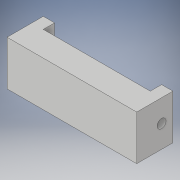
# Autodesk Inventor part: cap
Saved by Autodesk Inventor 2019 (Build 230136000, 136)
## iProperties
Created: 2019-05-07
Part Number: cap
Material: Generic
Document SubType Name: Modeling
Designer: Alex Jones
Density: 1 g/cm^3
Appearance: Default
Author: Alex Jones
Autodesk Inventor part; units mm, degrees
ref_plane "YZ Plane" through (0, 0, 0) normal (1, 0, 0) x (0, 1, 0)
ref_plane "XZ Plane" through (0, 0, 0) normal (0, 1, 0) x (-1, 0, 0)
ref_plane "XY Plane" through (0, 0, 0) normal (0, 0, 1) x (1, 0, 0)
sketch "Sketch1" plane through (0, 0, 0) normal (0, 0, 1) x (1, 0, 0)
  circle A0 centre (-40, 0) radius 2.5 projected
  arc A1 (-31.25, -10) -> (-30, -8.75) centre (-31.25, -8.75) ccw projected
  line L0 (-30, -3.6) -> (-30, -8.75) projected
  line L1 (-30.5, -3.1) -> (-30, -3.6) projected
  line L2 (-31.6, -3.1) -> (-30.5, -3.1) projected
  line L3 (-31.6, -5.5) -> (-31.6, -3.1) projected
  line L4 (-33.534, -5.5) -> (-31.6, -5.5) projected
  line L5 (-35.9, -3.134) -> (-33.534, -5.5) projected
  line L6 (-35.9, 3.134) -> (-35.9, -3.134) projected
  line L7 (-33.534, 5.5) -> (-35.9, 3.134) projected
  line L8 (-31.6, 5.5) -> (-33.534, 5.5) projected
  line L9 (-31.6, 3.1) -> (-31.6, 5.5) projected
  line L10 (-30.5, 3.1) -> (-31.6, 3.1) projected
  line L11 (-30, 3.6) -> (-30.5, 3.1) projected
  line L12 (-30, 8.75) -> (-30, 3.6) projected
  arc A2 (-30, 8.75) -> (-31.25, 10) centre (-31.25, 8.75) ccw projected
  line L13 (-36.4, 10) -> (-31.25, 10) projected
  line L14 (-36.9, 9.5) -> (-36.4, 10) projected
  line L15 (-36.9, 8.4) -> (-36.9, 9.5) projected
  line L16 (-34.5, 8.4) -> (-36.9, 8.4) projected
  line L17 (-34.5, 6.466) -> (-34.5, 8.4) projected
  line L18 (-36.866, 4.1) -> (-34.5, 6.466) projected
  line L19 (-43.134, 4.1) -> (-36.866, 4.1) projected
  line L20 (-45.5, 6.466) -> (-43.134, 4.1) projected
  line L21 (-45.5, 8.4) -> (-45.5, 6.466) projected
  line L22 (-43.1, 8.4) -> (-45.5, 8.4) projected
  line L23 (-43.1, 9.5) -> (-43.1, 8.4) projected
  line L24 (-43.6, 10) -> (-43.1, 9.5) projected
  line L25 (-48.75, 10) -> (-43.6, 10) projected
  arc A3 (-48.75, 10) -> (-50, 8.75) centre (-48.75, 8.75) ccw projected
  line L26 (-50, 3.6) -> (-50, 8.75) projected
  line L27 (-49.5, 3.1) -> (-50, 3.6) projected
  line L28 (-48.4, 3.1) -> (-49.5, 3.1) projected
  line L29 (-48.4, 5.5) -> (-48.4, 3.1) projected
  line L30 (-46.466, 5.5) -> (-48.4, 5.5) projected
  line L31 (-44.1, 3.134) -> (-46.466, 5.5) projected
  line L32 (-44.1, -3.134) -> (-44.1, 3.134) projected
  line L33 (-46.466, -5.5) -> (-44.1, -3.134) projected
  line L34 (-48.4, -5.5) -> (-46.466, -5.5) projected
  line L35 (-48.4, -3.1) -> (-48.4, -5.5) projected
  line L36 (-49.5, -3.1) -> (-48.4, -3.1) projected
  line L37 (-50, -3.6) -> (-49.5, -3.1) projected
  line L38 (-50, -8.75) -> (-50, -3.6) projected
  arc A4 (-50, -8.75) -> (-48.75, -10) centre (-48.75, -8.75) ccw projected
  line L39 (-43.6, -10) -> (-48.75, -10) projected
  line L40 (-43.1, -9.5) -> (-43.6, -10) projected
  line L41 (-43.1, -8.4) -> (-43.1, -9.5) projected
  line L42 (-45.5, -8.4) -> (-43.1, -8.4) projected
  line L43 (-45.5, -6.466) -> (-45.5, -8.4) projected
  line L44 (-43.134, -4.1) -> (-45.5, -6.466) projected
  line L45 (-36.866, -4.1) -> (-43.134, -4.1) projected
  line L46 (-34.5, -6.466) -> (-36.866, -4.1) projected
  line L47 (-34.5, -8.4) -> (-34.5, -6.466) projected
  line L48 (-36.9, -8.4) -> (-34.5, -8.4) projected
  line L49 (-36.9, -9.5) -> (-36.9, -8.4) projected
  line L50 (-36.4, -10) -> (-36.9, -9.5) projected
  line L51 (-31.25, -10) -> (-36.4, -10) projected
  circle A5 centre (0, 0) radius 2.5 projected
  arc A6 (8.75, -10) -> (10, -8.75) centre (8.75, -8.75) ccw projected
  line L52 (10, -3.6) -> (10, -8.75) projected
  line L53 (9.5, -3.1) -> (10, -3.6) projected
  line L54 (8.4, -3.1) -> (9.5, -3.1) projected
  line L55 (8.4, -5.5) -> (8.4, -3.1) projected
  line L56 (6.466, -5.5) -> (8.4, -5.5) projected
  line L57 (4.1, -3.134) -> (6.466, -5.5) projected
  line L58 (4.1, 3.134) -> (4.1, -3.134) projected
  line L59 (6.466, 5.5) -> (4.1, 3.134) projected
  line L60 (8.4, 5.5) -> (6.466, 5.5) projected
  line L61 (8.4, 3.1) -> (8.4, 5.5) projected
  line L62 (9.5, 3.1) -> (8.4, 3.1) projected
  line L63 (10, 3.6) -> (9.5, 3.1) projected
  line L64 (10, 8.75) -> (10, 3.6) projected
  arc A7 (10, 8.75) -> (8.75, 10) centre (8.75, 8.75) ccw projected
  line L65 (3.6, 10) -> (8.75, 10) projected
  line L66 (3.1, 9.5) -> (3.6, 10) projected
  line L67 (3.1, 8.4) -> (3.1, 9.5) projected
  line L68 (5.5, 8.4) -> (3.1, 8.4) projected
  line L69 (5.5, 6.466) -> (5.5, 8.4) projected
  line L70 (3.134, 4.1) -> (5.5, 6.466) projected
  line L71 (-3.134, 4.1) -> (3.134, 4.1) projected
  line L72 (-5.5, 6.466) -> (-3.134, 4.1) projected
  line L73 (-5.5, 8.4) -> (-5.5, 6.466) projected
  line L74 (-3.1, 8.4) -> (-5.5, 8.4) projected
  line L75 (-3.1, 9.5) -> (-3.1, 8.4) projected
  line L76 (-3.6, 10) -> (-3.1, 9.5) projected
  line L77 (-8.75, 10) -> (-3.6, 10) projected
  arc A8 (-8.75, 10) -> (-10, 8.75) centre (-8.75, 8.75) ccw projected
  line L78 (-10, 3.6) -> (-10, 8.75) projected
  line L79 (-9.5, 3.1) -> (-10, 3.6) projected
  line L80 (-8.4, 3.1) -> (-9.5, 3.1) projected
  line L81 (-8.4, 5.5) -> (-8.4, 3.1) projected
  line L82 (-6.466, 5.5) -> (-8.4, 5.5) projected
  line L83 (-4.1, 3.134) -> (-6.466, 5.5) projected
  line L84 (-4.1, -3.134) -> (-4.1, 3.134) projected
  line L85 (-6.466, -5.5) -> (-4.1, -3.134) projected
  line L86 (-8.4, -5.5) -> (-6.466, -5.5) projected
  line L87 (-8.4, -3.1) -> (-8.4, -5.5) projected
  line L88 (-9.5, -3.1) -> (-8.4, -3.1) projected
  line L89 (-10, -3.6) -> (-9.5, -3.1) projected
  line L90 (-10, -8.75) -> (-10, -3.6) projected
  arc A9 (-10, -8.75) -> (-8.75, -10) centre (-8.75, -8.75) ccw projected
  line L91 (-3.6, -10) -> (-8.75, -10) projected
  line L92 (-3.1, -9.5) -> (-3.6, -10) projected
  line L93 (-3.1, -8.4) -> (-3.1, -9.5) projected
  line L94 (-5.5, -8.4) -> (-3.1, -8.4) projected
  line L95 (-5.5, -6.466) -> (-5.5, -8.4) projected
  line L96 (-3.134, -4.1) -> (-5.5, -6.466) projected
  line L97 (3.134, -4.1) -> (-3.134, -4.1) projected
  line L98 (5.5, -6.466) -> (3.134, -4.1) projected
  line L99 (5.5, -8.4) -> (5.5, -6.466) projected
  line L100 (3.1, -8.4) -> (5.5, -8.4) projected
  line L101 (3.1, -9.5) -> (3.1, -8.4) projected
  line L102 (3.6, -10) -> (3.1, -9.5) projected
  line L103 (8.75, -10) -> (3.6, -10) projected
  line L104 (-50, -10) -> (-50, 10)
  line L105 (10, 10) -> (10, -10)
  line L106 (-30, -10) -> (-30, 10)
  line L107 (-10, 10) -> (-10, -10)
  line L108 (-52.54, -12.54) -> (12.54, -12.54)
  line L109 (12.54, -12.54) -> (12.54, 12.54)
  line L110 (12.54, 12.54) -> (-52.54, 12.54)
  line L111 (-52.54, 12.54) -> (-52.54, -12.54)
  line L112 (10, -10) -> (-10, -10)
  line L113 (-30, -10) -> (-50, -10)
  line L114 (-50, 10) -> (-30, 10)
  line L115 (-10, 10) -> (10, 10)
  point P0 (0, 0)
  constraints: 24 end point, 8 parallel, 3 perpendicular, 2 horizontal, 1 point on line
extrude "Extrusion1" add sketch "Sketch1" against normal blind 7.62 contours L111 L110 L109 L108
sketch "Sketch2" plane through (0, 0, 0) normal (0, 0, 1) x (1, 0, 0)
  line L0 (-52.54, -12.54) -> (-52.54, 12.54) projected
  line L1 (12.54, -12.54) -> (12.54, 12.54) projected
  line L2 (-52.54, -12.54) -> (12.54, -12.54)
  line L3 (12.54, -12.54) -> (12.54, 12.54)
  line L4 (12.54, 12.54) -> (-52.54, 12.54)
  line L5 (-52.54, 12.54) -> (-52.54, -12.54)
  point P0 (0, 0)
  constraints: 8 end point, 2 parallel, 1 horizontal, 1 perpendicular
extrude "Extrusion2" add sketch "Sketch2" along normal blind 6.35
sketch "Sketch3" plane through (12.54, -12.54, -7.62) normal (1, 0, 0) x (0, 0, -1)
  line L0 (0, 0) -> (-13.97, 0) projected
  line L1 (0, 25.08) -> (0, 0) projected
  line L2 (0, 25.08) -> (-13.97, 25.08) projected
  line L3 (-13.97, 0) -> (-13.97, 25.08) projected
  point P0 (-7.62, 12.54)
extrude "Extrusion3" add sketch "Sketch3" along normal blind 3.81
sketch "Sketch4" plane through (-52.54, -12.54, -7.62) normal (-1, 0, 0) x (0, 0, 1)
  line L0 (0, 25.08) -> (13.97, 25.08) projected
  line L1 (0, 0) -> (0, 25.08) projected
  line L2 (13.97, 0) -> (0, 0) projected
  line L3 (13.97, 25.08) -> (13.97, 0) projected
  point P0 (7.62, 12.54)
extrude "Extrusion4" add sketch "Sketch4" along normal blind 3.81
sketch "Sketch5" plane through (0, 0, -7.62) normal (0, 0, -1) x (-1, 0, 0)
  line L0 (-16.35, -12.54) -> (-16.35, 12.54) projected
  line L1 (56.35, -12.54) -> (-16.35, -12.54) projected
  line L2 (-16.35, 12.54) -> (-10, 12.54)
  line L3 (-10, 12.54) -> (-10, -12.54)
  line L4 (-10, -12.54) -> (-16.35, -12.54)
  line L5 (-16.35, -12.54) -> (-16.35, 12.54)
  line L6 (56.35, 12.54) -> (50, 12.54)
  line L7 (50, 12.54) -> (50, -12.54)
  line L8 (50, -12.54) -> (56.35, -12.54)
  line L9 (56.35, -12.54) -> (56.35, 12.54)
  line L10 (50, 10) -> (50, -10) projected
  line L11 (-10, -10) -> (-10, 10) projected
  point P0 (0, 0)
  dimension "d10" = 0
  dimension "d11" = 0
  constraints: 16 end point, 4 parallel, 2 horizontal, 2 perpendicular, 2 point on line
  measures "d10" distance between parallel lines of L10 L7
  measures "d11" distance between parallel lines of L11 L3
extrude "Extrusion5" add sketch "Sketch5" along normal blind 6.35
sketch "Sketch6" plane through (-56.35, -12.54, -7.62) normal (-1, 0, 0) x (0, 0, 1)
  line L0 (13.97, 25.08) -> (-6.35, 25.08) projected
  line L1 (0, 0) -> (-6.35, 0) projected
  circle A0 centre (0, 12.54) radius 2.5
  line L2 (13.97, 25.08) -> (-6.35, 25.08) projected
  line L3 (0, 25.08) -> (0, -0.7911)
  line L4 (-6.35, 0) -> (-6.35, 25.08) projected
  point P0 (7.62, 12.54)
  dimension "d14" = 5
  dimension "d19" = 6.35
  constraints: 2 end point, 2 point on line, 1 centre point, 1 perpendicular
  measures "d14" diameter of A0
  measures "d19" distance between parallel lines of L4 L3
extrude "Extrusion6" cut sketch "Sketch6" against normal through all contours L3 A0 | A0 L3
sketch "Sketch8" plane through (-10, -10, 0) normal (1, 0, 0) x (0, 0, -1)
  arc A0 (7.62, 12.5) -> (7.62, 7.5) centre (7.62, 10) ccw projected
  line L0 (7.62, 7.5) -> (7.62, 0) projected
  line L1 (7.62, 12.5) -> (7.62, 7.5)
  point P0 (0, 10)
  constraints: 2 end point, 1 vertical
extrude "Extrusion7" add sketch "Sketch8" against normal up to surface (20 mm away)
body "Solid1"
